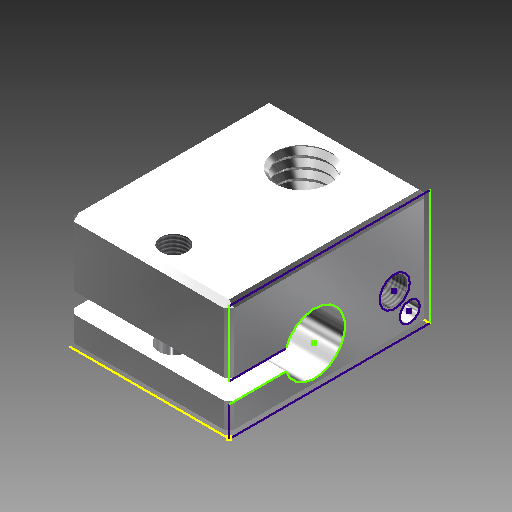
# Autodesk Inventor part: heater
Saved by Autodesk Inventor 2018 (Build 220112000, 112)
## iProperties
Created: 2015-02-05
Part Number: heater
Material: Aluminium 6061
Document SubType Name: Modeling
Designer: Parabolik
Density: 2.7 g/cm^3
Appearance: Aluminium - flach
Author: Parabolik
Autodesk Inventor part; units mm, degrees
ref_plane "YZ Plane" through (0, 0, 0) normal (1, 0, 0) x (0, 1, 0)
ref_plane "XZ Plane" through (0, 0, 0) normal (0, 1, 0) x (-1, 0, 0)
sketch "Эскиз1" plane through (0, 0, 0) normal (1, 0, 0) x (0, 1, 0)
  arc A0 (3, -5.6451) -> (5, -5.6451) centre (4, -8.5) ccw
  line L0 (5, 0) -> (5, -5.6451)
  line L1 (0, -20) -> (0, 0)
  line L2 (11.5, 0) -> (11.5, -20)
  line L3 (11.5, -20) -> (0, -20)
  line L4 (3, -5.6451) -> (3, 0)
  line L5 (3, 0) -> (0, 0)
  line L6 (11.5, 0) -> (5, 0)
  dimension "d4" = 3.025
  dimension "d6" = 11.5
  dimension "d8" = 20
  dimension "d9" = 6.5
  dimension "d10" = 8.5
  dimension "d11" = 4
  constraints: 14 end point, 2 horizontal, 2 point on circle, 2 vertical, 1 centre point, 1 coincident, 1 perpendicular
  measures "d4" radius of A0
  measures "d6" distance between parallel lines of L1 L2
  measures "d8" distance between parallel lines of L6 L3
  measures "d9" distance between parallel lines of L0 L2
  measures "d10" distance from line of L6 A0.centre
  measures "d11" distance from line of L1 A0.centre
extrude "Выдавливание1" add sketch "Эскиз1" against normal blind 16
sketch "Эскиз2" plane through (0, 0, 0) normal (1, 0, 0) x (0, 0, -1)
  circle A0 centre (18, 2) radius 1
  circle A1 centre (16.5, 4.5) radius 1.5
  line L0 (20, 0) -> (0, 0) projected
  line L1 (20, 11.5) -> (20, 0) projected
  dimension "d14" = 2
  dimension "d15" = 3
  dimension "d16" = 2
  dimension "d17" = 2
  dimension "d18" = 3.5
  dimension "d19" = 4.5
  constraints: 2 centre point
  measures "d14" diameter of A0
  measures "d15" diameter of A1
  measures "d16" distance from line of A0.centre L0
  measures "d17" distance from line of A0.centre L1
  measures "d18" distance from line of L1 A1.centre
  measures "d19" distance from line of A1.centre L0
hole "Отверстие1" at (0, 4.5, -16.5) direction (-1, 0, 0) diameter 2.621 depth 4 tip angle 118 thread size "M3x0.35" class "6H" standard "ISO Metric profile"
hole "Отверстие3" at (0, 2, -18) direction (-1, 0, 0) diameter 1.2 depth 4.5 tip angle 118
hole "Отверстие4" at (0, 2, -18) direction (-1, 0, 0) diameter 2 depth 2 tip angle 118
sketch "Эскиз3" plane through (0, 0, -20) normal (0, -1, 0) x (1, 0, 0)
  circle A0 centre (-8, 17.5) radius 1.5
  line L0 (0, 0) -> (0, 20) projected
  line L1 (0, 0) -> (-16, 0) projected
  line L2 (0, 20) -> (-16, 20) projected
  circle A1 centre (-8, 4.5) radius 2.5
  dimension "d31" = 3
  dimension "d32" = 8
  dimension "d34" = 2.5
  dimension "d35" = 5
  dimension "d36" = 4.5
  dimension "d37" = 8
  constraints: 2 centre point
  measures "d31" diameter of A0
  measures "d32" distance from line of A0.centre L0
  measures "d34" distance from line of A0.centre L2
  measures "d35" diameter of A1
  measures "d36" distance from line of A1.centre L1
  measures "d37" distance from line of A1.centre L0
hole "Отверстие2" at (-8, 0, -2.5) direction (0, 1, 0) diameter 2.621 depth 11.5 counterbore diameter 3.023 counterbore depth 5 thread size "M3x0.35" class "6H" standard "ISO Metric profile"
extrude "Выдавливание4" cut sketch "Эскиз3" against normal blind 12 contours A1
chamfer "Фаска1" distance 0.5 angle 45 14 edges at (0, 11.5, -10) (-8, 11.5, -20) (-16, 11.5, -10) (-8, 11.5, 0) (0, 5.75, -20) (-16, 5.75, -20) (-8, 0, -20) (-16, 8.25, 0) (-16, 1.5, 0) (-16, 0, -10) (0, 8.25, 0) (0, 1.5, 0) (-8, 0, 0) (0, 0, -10)
ref_plane "РабПлоскость2" through (-0.5, 0.5, -15.5) normal (0, 0, -1) x (-1, 0, 0)
sketch "Эскиз5" plane through (-0.5, 0.5, -15.5) normal (0, 0, -1) x (-1, 0, 0)
  line L0 (6.1895, 11) -> (8.8105, 11) projected
  line L1 (7.5, 11) -> (7.5, -1.8215)
  line L2 (10, -0.5) -> (5, -0.5) projected
  line L3 (10, -0.5) -> (10.8, -0.5)
  line L4 (15, -0.5) -> (0, -0.5) projected
  line L5 (10, -0.5) -> (10, -1.4)
  line L6 (10.5, -0.9) -> (10, -0.5)
  line L7 (10.5, -0.9) -> (10.5, -1)
  line L8 (10.5, -1) -> (10, -1.4)
  point P0 (-0.5, -0.5)
  dimension "d84" = 0.8
  dimension "d85" = 0.9
  dimension "d88" = 0.1
  dimension "d89" = 0.4
  constraints: 13 end point, 3 vertical, 1 midpoint, 1 point on line
  measures "d84" distance of L2.start L3.end
  measures "d85" distance of L2.start L5.end
  measures "d88" distance of L6.start L7.end
  measures "d89" vertical distance of L6.start L2.start
coil "Пружина2" sketch "Эскиз5" operation cut axis through (-8, 11.5, -15.5) along (0, 1, 0) pitch 1 turns 12.5 hand right
